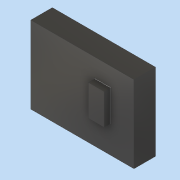
# Autodesk Inventor part: 激光传感器模型
Saved by Autodesk Inventor 2019 (Build 230136000, 136)
## iProperties
Created: 2020-10-24
Part Number: 激光传感器模型
Material: 氮化硅
Document SubType Name: Modeling
Designer: Wang Hua
Density: 3.18 g/cm^3
Appearance: 铬 - 黑色抛光
Author: Wang Hua
Autodesk Inventor part; units mm, degrees
ref_plane "YZ Plane" through (0, 0, 0) normal (1, 0, 0) x (0, 1, 0)
ref_plane "XZ Plane" through (0, 0, 0) normal (0, 1, 0) x (-1, 0, 0)
ref_plane "XY Plane" through (0, 0, 0) normal (0, 0, 1) x (1, 0, 0)
sketch "草图1" plane through (0, 0, 0) normal (0, 0, 1) x (1, 0, 0)
  line L0 (8.15, -6.1) -> (-8.15, -6.1)
  line L1 (-8.15, -6.1) -> (-8.15, 6.1)
  line L2 (-8.15, 6.1) -> (8.15, 6.1)
  line L3 (8.15, 6.1) -> (8.15, -6.1)
  line L4 (8.15, -6.1) -> (-8.15, 6.1) construction
  line L5 (-8.15, -6.1) -> (8.15, 6.1) construction
  point P0 (0, 0)
  dimension "d0" = 16.3
  dimension "d1" = 12.2
  constraints: 12 end point, 2 midpoint, 2 parallel, 1 horizontal, 1 perpendicular
  measures "d0" distance between parallel lines of L3 L1
  measures "d1" distance between parallel lines of L0 L2
extrude "拉伸1" add sketch "草图1" along normal blind 3.4
sketch "草图2" plane through (0, 0, 3.4) normal (0, 0, 1) x (1, 0, 0)
  line L0 (4.45, 0) -> (4.45, 4.1654) construction
  line L1 (8.15, 6.1) -> (8.15, -6.1) construction
  line L2 (4.45, 3.1034) -> (1.95, 3.1034)
  line L3 (1.95, 3.1034) -> (1.95, -1.7966)
  line L4 (1.95, -1.7966) -> (4.45, -1.7966)
  line L5 (4.45, -1.7966) -> (4.45, 3.1034)
  point P0 (0, 0)
  dimension "d4" = 3.7
  dimension "d5" = 4.9
  dimension "d6" = 2.5
  constraints: 10 end point, 2 parallel, 1 horizontal, 1 perpendicular, 1 point on line, 1 vertical
  measures "d4" distance between parallel lines of L1 L0
  measures "d5" distance of L2.end L3.end
  measures "d6" distance of L2.start L2.end
extrude "拉伸2" add sketch "草图2" along normal blind 1
fillet "圆角1" radius 0.1 4 edges at (4.45, 0.6534, 3.4) (3.2, 3.1034, 3.4) (3.2, -1.7966, 3.4) (1.95, 0.6534, 3.4)
